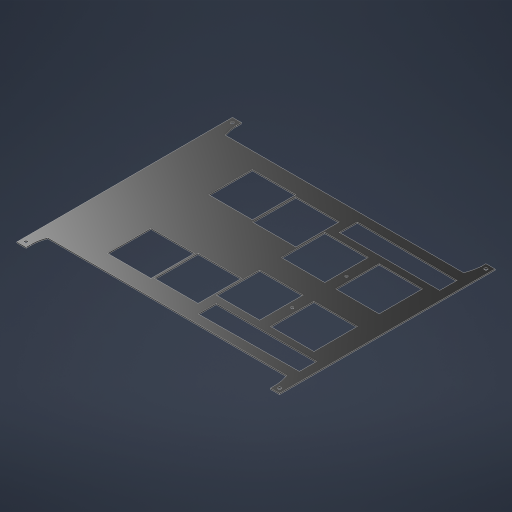
# Autodesk Inventor part: belly pan
Saved by Autodesk Inventor 2024 (Build 280153000, 153)
## iProperties
Created: 2023-12-20
Part Number: belly pan
Material: Generic
Document SubType Name: Modeling
Designer: elite
Density: 1 g/cm^3
Appearance: Glossy - Black
Author: elite
Autodesk Inventor part; units mm, degrees
ref_plane "YZ Plane" through (0, 0, 0) normal (1, 0, 0) x (0, 1, 0)
ref_plane "XZ Plane" through (0, 0, 0) normal (0, 1, 0) x (-1, 0, 0)
ref_plane "XY Plane" through (0, 0, 0) normal (0, 0, 1) x (1, 0, 0)
sketch "Sketch1" plane through (0, 0, 0) normal (0, 1, 0) x (-1, 0, 0)
  line L0 (0, 0) -> (355.6, 0)
  line L1 (355.6, 0) -> (355.6, -289.56)
  line L2 (355.6, -289.56) -> (0, -289.56)
  line L3 (0, -289.56) -> (0, 0)
  circle A0 centre (355.6, 0) radius 2.1082
  line L4 (355.6, 0) -> (361.95, 0)
  line L5 (355.6, 0) -> (355.6, 6.35)
  line L6 (355.6, 6.35) -> (361.95, 6.35)
  line L7 (0, -289.56) -> (0, -295.91)
  line L8 (0, -295.91) -> (-6.35, -295.91)
  line L9 (-6.35, -295.91) -> (361.95, -295.91)
  line L10 (361.95, -295.91) -> (361.95, 6.35)
  line L11 (361.95, 6.35) -> (-6.35, 6.35)
  line L12 (-6.35, 6.35) -> (-6.35, -295.91)
  circle A1 centre (355.6, -289.56) radius 2.1082
  circle A2 centre (0, -289.56) radius 2.1082
  circle A3 centre (0, 0) radius 2.1082
  line L13 (0, 0) -> (0, -20.32)
  line L14 (0, -20.32) -> (10.16, -20.32)
  line L15 (0, 0) -> (5.08, 0)
  line L16 (0, -289.56) -> (5.08, -289.56)
  line L17 (0, -289.56) -> (0, -269.24)
  line L18 (0, -269.24) -> (11.0826, -269.24)
  line L19 (355.6, 0) -> (355.6, -20.32)
  line L20 (355.6, -20.32) -> (345.44, -20.32)
  line L21 (355.6, 0) -> (350.52, 0)
  line L22 (355.6, -289.56) -> (350.52, -289.56)
  line L23 (355.6, -289.56) -> (355.6, -269.24)
  line L24 (355.6, -269.24) -> (345.44, -269.24)
  line L25 (345.44, -20.32) -> (10.16, -20.32)
  line L26 (355.6, -20.32) -> (355.6, -33.02)
  line L27 (355.6, -33.02) -> (0, -33.02)
  line L28 (355.6, -269.24) -> (355.6, -256.54)
  line L29 (355.6, -256.54) -> (0, -256.54)
  line L30 (345.44, -269.24) -> (11.0826, -269.24)
  line L31 (0, 0) -> (6.35, 0)
  arc A4 (6.35, 0) -> (10.16, -20.32) centre (82.4575, 3.753) ccw
  line L32 (6.35, 0) -> (-6.35, 0)
  line L33 (-6.35, 0) -> (-6.35, -289.56)
  line L34 (-6.35, -289.56) -> (6.35, -289.56)
  line L35 (6.35, -289.56) -> (6.35, 0)
  arc A5 (11.0826, -269.24) -> (6.35, -289.56) centre (82.2313, -296.5221) ccw
  line L36 (355.6, 0) -> (349.25, 0)
  line L37 (349.25, 0) -> (349.25, -289.56)
  arc A6 (349.25, -289.56) -> (345.44, -269.24) centre (298.4597, -288.566) ccw
  arc A7 (345.44, -20.32) -> (349.25, 0) centre (298.4597, -0.994) ccw
  line L38 (349.25, 0) -> (349.25, 6.35)
  line L39 (349.25, -289.56) -> (349.25, -295.91)
  line L40 (6.35, -289.56) -> (6.35, -295.91)
  line L41 (6.35, 0) -> (6.35, 6.35)
  dimension "d0" = 355.6
  dimension "d1" = 289.56
  dimension "d2" = 4.2164
  dimension "d3" = 6.35
  dimension "d4" = 6.35
  dimension "d5" = 6.35
  dimension "d6" = 6.35
  dimension "d7" = 20.32
  dimension "d8" = 10.16
  dimension "d10" = 20.32
  dimension "d12" = 20.32
  dimension "d13" = 10.16
  dimension "d16" = 5.08
  dimension "d17" = 20.32
  dimension "d18" = 10.16
  dimension "d20" = 12.7
  dimension "d21" = 12.7
  dimension "d23" = 6.35
  dimension "d24" = 76.2
  dimension "d25" = 76.2
  dimension "d26" = 6.35
  dimension "d27" = 50.8
  dimension "d28" = 50.8
  constraints: 84 end point, 21 point on line, 14 perpendicular, 8 centre point, 8 point on circle, 6 parallel, 5 horizontal, 4 coincident, 2 vertical
  measures "d0" distance of L1.end L2.end
  measures "d1" distance of L2.end L0.start
  measures "d2" diameter of A0
  measures "d3" distance of L4.start L4.end
  measures "d4" distance of L4.start L5.end
  measures "d5" distance of L2.end L7.end
  measures "d6" distance of L7.end L8.end
  measures "d7" distance of L13.start L13.end
  measures "d8" distance of L13.end L14.end
  measures "d10" distance of L16.start L17.end
  measures "d12" distance of L4.start L19.end
  measures "d13" distance of L19.end L20.end
  measures "d16" distance of L22.start L22.end
  measures "d17" distance of L22.start L23.end
  measures "d18" distance of L23.end L24.end
  measures "d20" distance of L19.end L26.end
  measures "d21" distance of L23.end L28.end
  measures "d23" distance of L13.start L31.end
  measures "d24" radius of A4
  measures "d25" radius of A5
  measures "d26" distance of L4.start L36.end
  measures "d27" radius of A6
  measures "d28" radius of A7
extrude "Extrusion1" add sketch "Sketch1" along normal blind 1.5875 contours A3 L32 L12 L11 L41 L0 | L0 L35 L14 L3 A3 | L3 A2 L34 L12 L32 A3 | L14 L35 L27 L3 | A4 L14 L35 | L27 L35 L29 L3 | L14 L25 L20 L37 L27 L35 | L34 A2 L7 L8 L12 | L38 L11 L5 A0 L0 | L0 A0 L1 L20 L37 A7 | L29 L35 L18 L3 | L27 L37 L29 L35 | L37 L20 A7 | L18 L35 L2 A2 L3 | L29 L37 L24 L30 L18 L35 | L37 L20 L1 L27 | L27 L1 L29 L37 | L7 A2 L2 L40 L9 | L6 L10 L4 A0 L5 | L18 A5 L35 | L29 L1 L24 L37 | L1 A0 L4 L10 L9 L39 L2 A1 | L37 A6 L24 | L24 L1 A1 L2 A6 L37
sketch "Sketch2" plane through (0, 1.5875, 0) normal (0, 1, 0) x (1, 0, 0)
  circle A0 centre (-355.6, 289.56) radius 2.1082 projected
  line L0 (-355.6, 289.56) -> (-355.6, 246.38)
  line L1 (-355.6, 246.38) -> (-284.48, 246.38)
  line L2 (-355.6, 289.56) -> (-355.6, 185.42)
  line L3 (-355.6, 185.42) -> (-223.52, 185.42)
  line L4 (-284.48, 246.38) -> (-223.52, 246.38)
  line L5 (-223.52, 246.38) -> (-223.52, 185.42)
  line L6 (-223.52, 185.42) -> (-284.48, 185.42)
  line L7 (-284.48, 185.42) -> (-284.48, 246.38)
  line L8 (-355.6, 289.56) -> (-355.6, 243.84)
  line L9 (-355.6, 243.84) -> (-220.98, 243.84)
  line L10 (-355.6, 289.56) -> (-355.6, 184.15)
  line L11 (-355.6, 289.56) -> (-355.6, 182.88)
  line L12 (-355.6, 182.88) -> (-160.02, 182.88)
  line L13 (-220.98, 243.84) -> (-160.02, 243.84)
  line L14 (-160.02, 243.84) -> (-160.02, 182.88)
  line L15 (-160.02, 182.88) -> (-220.98, 182.88)
  line L16 (-220.98, 182.88) -> (-220.98, 243.84)
  line L17 (-355.6, 289.56) -> (-355.6, 220.98)
  line L18 (-355.6, 220.98) -> (-157.48, 220.98)
  line L19 (-355.6, 289.56) -> (-355.6, 160.02)
  line L20 (-355.6, 160.02) -> (-96.52, 160.02)
  line L21 (-157.48, 220.98) -> (-96.52, 220.98)
  line L22 (-96.52, 220.98) -> (-96.52, 160.02)
  line L23 (-96.52, 160.02) -> (-157.48, 160.02)
  line L24 (-157.48, 160.02) -> (-157.48, 220.98)
  line L25 (-355.6, 289.56) -> (-81.28, 289.56)
  line L26 (-81.28, 289.56) -> (-81.28, 220.98)
  line L27 (-355.6, 289.56) -> (-20.32, 289.56)
  line L28 (-20.32, 289.56) -> (-20.32, 160.02)
  line L29 (-81.28, 220.98) -> (-20.32, 220.98)
  line L30 (-20.32, 220.98) -> (-20.32, 160.02)
  line L31 (-20.32, 160.02) -> (-81.28, 160.02)
  line L32 (-81.28, 160.02) -> (-81.28, 220.98)
  line L33 (-355.6, 289.56) -> (-160.02, 289.56)
  line L34 (-160.02, 289.56) -> (-160.02, 269.24)
  line L35 (-11.0826, 269.24) -> (-345.44, 269.24) projected
  line L36 (-160.02, 269.24) -> (-160.02, 256.54)
  line L37 (-160.02, 256.54) -> (6.35, 255.27)
  line L38 (6.35, -6.35) -> (6.35, 295.91) projected
  line L39 (6.35, 255.27) -> (-6.3496, 255.3669)
  line L40 (-160.02, 289.56) -> (-160.02, 231.14)
  line L41 (-6.3496, 255.3669) -> (-6.3496, 231.14)
  line L42 (-6.3496, 231.14) -> (-160.02, 231.14)
  line L43 (-160.02, 256.54) -> (-147.32, 256.54)
  line L44 (-147.32, 256.54) -> (-147.32, 231.14)
  line L45 (-147.32, 231.14) -> (-160.02, 231.14)
  line L46 (-160.02, 231.14) -> (-160.02, 256.54)
  line L47 (6.35, 295.91) -> (6.35, -6.35)
  line L48 (-361.95, 295.91) -> (-361.95, -6.35) projected
  line L49 (6.35, 144.78) -> (-361.95, 144.78)
  circle A1 centre (-355.6, 0) radius 2.1082
  line L50 (-355.6, 0) -> (-355.6, 43.18)
  line L51 (-355.6, 43.18) -> (-284.48, 43.18)
  line L52 (-355.6, 0) -> (-355.6, 104.14)
  line L53 (-355.6, 104.14) -> (-223.52, 104.14)
  line L54 (-284.48, 43.18) -> (-223.52, 43.18)
  line L55 (-223.52, 43.18) -> (-223.52, 104.14)
  line L56 (-223.52, 104.14) -> (-284.48, 104.14)
  line L57 (-284.48, 104.14) -> (-284.48, 43.18)
  line L58 (-355.6, 0) -> (-355.6, 45.72)
  line L59 (-355.6, 45.72) -> (-220.98, 45.72)
  line L60 (-355.6, 0) -> (-355.6, 105.41)
  line L61 (-355.6, 0) -> (-355.6, 106.68)
  line L62 (-355.6, 106.68) -> (-160.02, 106.68)
  line L63 (-220.98, 45.72) -> (-160.02, 45.72)
  line L64 (-160.02, 45.72) -> (-160.02, 106.68)
  line L65 (-160.02, 106.68) -> (-220.98, 106.68)
  line L66 (-220.98, 106.68) -> (-220.98, 45.72)
  line L67 (-355.6, 0) -> (-355.6, 68.58)
  line L68 (-355.6, 68.58) -> (-157.48, 68.58)
  line L69 (-355.6, 0) -> (-355.6, 129.54)
  line L70 (-355.6, 129.54) -> (-96.52, 129.54)
  line L71 (-157.48, 68.58) -> (-96.52, 68.58)
  line L72 (-96.52, 68.58) -> (-96.52, 129.54)
  line L73 (-96.52, 129.54) -> (-157.48, 129.54)
  line L74 (-157.48, 129.54) -> (-157.48, 68.58)
  line L75 (-355.6, 0) -> (-81.28, 0)
  line L76 (-81.28, 0) -> (-81.28, 68.58)
  line L77 (-355.6, 0) -> (-20.32, 0)
  line L78 (-20.32, 0) -> (-20.32, 129.54)
  line L79 (-81.28, 68.58) -> (-20.32, 68.58)
  line L80 (-20.32, 68.58) -> (-20.32, 129.54)
  line L81 (-20.32, 129.54) -> (-81.28, 129.54)
  line L82 (-81.28, 129.54) -> (-81.28, 68.58)
  line L83 (-355.6, 0) -> (-160.02, 0)
  line L84 (-160.02, 0) -> (-160.02, 20.32)
  line L85 (-11.0826, 20.32) -> (-345.44, 20.32)
  line L86 (-160.02, 20.32) -> (-160.02, 33.02)
  line L87 (-160.02, 33.02) -> (6.35, 34.29)
  line L88 (6.35, 34.29) -> (-6.3496, 34.1931)
  line L89 (-160.02, 0) -> (-160.02, 58.42)
  line L90 (-6.3496, 34.1931) -> (-6.3496, 58.42)
  line L91 (-6.3496, 58.42) -> (-160.02, 58.42)
  line L92 (-160.02, 33.02) -> (-147.32, 33.02)
  line L93 (-147.32, 33.02) -> (-147.32, 58.42)
  line L94 (-147.32, 58.42) -> (-160.02, 58.42)
  line L95 (-160.02, 58.42) -> (-160.02, 33.02)
  line L96 (-361.95, -6.35) -> (-361.95, 295.91)
  line L97 (-96.52, 160.02) -> (-81.28, 160.02)
  line L98 (-88.9, 160.02) -> (-88.9, 144.78)
  line L99 (-88.9, 144.78) -> (-88.9, 182.88)
  circle A2 centre (-88.9, 182.88) radius 1.778
  line L100 (-88.9, 144.78) -> (-88.9, 106.68)
  circle A3 centre (-88.9, 106.68) radius 1.778
  point P0 (0, 0)
  point P1 (-223.52, 243.84)
  point P2 (-284.48, 243.84)
  point P3 (-147.32, 256.4431)
  point P4 (-147.32, 33.1169)
  dimension "d31" = 43.18
  dimension "d32" = 71.12
  dimension "d33" = 104.14
  dimension "d34" = 132.08
  dimension "d35" = 45.72
  dimension "d36" = 134.62
  dimension "d37" = 105.41
  dimension "d38" = 106.68
  dimension "d39" = 195.58
  dimension "d42" = 68.58
  dimension "d43" = 198.12
  dimension "d44" = 129.54
  dimension "d45" = 259.08
  dimension "d46" = 274.32
  dimension "d47" = 68.58
  dimension "d49" = 335.28
  dimension "d50" = 129.54
  dimension "d51" = 195.58
  dimension "d52" = 12.7
  dimension "d53" = 12.7
  dimension "d54" = 58.42
  dimension "d55" = 12.7
  dimension "d56" = 38.1
  dimension "d57" = 3.556
  dimension "d58" = 38.1
  dimension "d59" = 3.556
  constraints: 196 end point, 40 symmetric about line, 29 point on line, 13 perpendicular, 12 parallel, 6 horizontal, 5 vertical, 3 centre point, 3 midpoint, 2 coincident, 1 other
  measures "d31" distance of L0.start L0.end
  measures "d32" distance of L0.end L1.end
  measures "d33" distance of L0.start L2.end
  measures "d34" distance of L2.end L3.end
  measures "d35" distance of L0.start L8.end
  measures "d36" distance of L8.end L9.end
  measures "d37" distance of L0.start L10.end
  measures "d38" distance of L0.start L11.end
  measures "d39" distance of L11.end L12.end
  measures "d42" distance of L0.start L17.end
  measures "d43" distance of L17.end L18.end
  measures "d44" distance of L0.start L19.end
  measures "d45" distance of L19.end L20.end
  measures "d46" distance of L0.start L25.end
  measures "d47" distance of L25.end L26.end
  measures "d49" distance of L0.start L27.end
  measures "d50" distance of L27.end L28.end
  measures "d51" distance of L0.start L33.end
  measures "d52" distance of L34.end L36.end
  measures "d53" distance of L37.end L39.end
  measures "d54" distance of L33.end L40.end
  measures "d55" distance of L44.end L45.end
  measures "d56" distance of L98.end L99.end
  measures "d57" diameter of A2
  measures "d58" distance of L98.end L100.end
  measures "d59" diameter of A3
extrude "Extrusion2" cut sketch "Sketch2" against normal blind 25.4 contours L87 L78 L91 L90 | A3 | L4 L5 L9 L7 | L9 L5 L18 L7 | L37 L28 L42 L26 | L26 L42 L44 L37 | L14 L18 L16 L13 | L18 L5 L3 L7 | A2 | L37 L41 L42 L28 | L29 L28 L31 L32 | L18 L14 L12 L16 | L21 L22 L20 L24 | L87 L76 L91 L78 | L87 L93 L91 L76 | L79 L82 L81 L78 | L64 L63 L66 L68 | L68 L66 L62 L64 | L74 L70 L72 L71 | L59 L57 L68 L55 | L55 L54 L57 L59 | L68 L57 L53 L55
body "Solid1"
